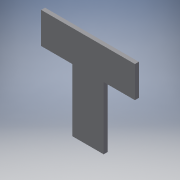
# Autodesk Inventor part: Frame T Gussets
Saved by Autodesk Inventor 2017 (Build 210142000, 142)
## iProperties
Created: 2017-12-29
Part Number: Frame T Gussets
Material: Generic
Document SubType Name: Modeling
Designer: anikasoojin
Density: 1 g/cm^3
Appearance: Default
Author: anikasoojin
Autodesk Inventor part; units mm, degrees
ref_plane "YZ Plane" through (0, 0, 0) normal (1, 0, 0) x (0, 1, 0)
ref_plane "XZ Plane" through (0, 0, 0) normal (0, 1, 0) x (-1, 0, 0)
ref_plane "XY Plane" through (0, 0, 0) normal (0, 0, 1) x (1, 0, 0)
sketch "Sketch1" plane through (0, 0, 0) normal (0, 0, 1) x (1, 0, 0)
  line L0 (-18.0361, 37.9933) -> (2.0277, 37.9933)
  line L1 (6.0832, 12.5933) -> (6.0832, -38.2067)
  line L2 (6.0832, -38.2067) -> (-19.3168, -38.2067)
  line L3 (-19.3168, -38.2067) -> (-19.3168, 12.5933)
  line L4 (-44.7168, 37.9933) -> (31.4832, 37.9933)
  line L5 (31.4832, 37.9933) -> (31.4832, 12.5933)
  line L6 (-44.7168, 12.5933) -> (-44.7168, 37.9933)
  line L7 (31.4832, 12.5933) -> (6.0832, 12.5933)
  line L8 (-19.3168, 12.5933) -> (-44.7168, 12.5933)
  point P0 (0, 0)
  dimension "d0" = 76.2
  dimension "d1" = 25.4
  dimension "d2" = 25.4
  dimension "d3" = 25.4
  dimension "d4" = 50.8
  dimension "d5" = 25.4
  constraints: 18 end point, 5 parallel, 2 horizontal, 2 perpendicular, 1 point on line
  measures "d0" distance between parallel lines of L5 L6
  measures "d1" distance of L1.end L2.end
  measures "d2" distance of L4.end L5.end
  measures "d3" distance of L6.start L4.start
  measures "d4" distance of L1.start L1.end
  measures "d5" distance of L3.end L6.start
extrude "Extrusion1" add sketch "Sketch1" along normal blind 3.175
fillet "Fillet1" radius 3.175 3 edges at (-44.7168, 12.5933, 1.5875) (-19.3168, 12.5933, 1.5875) (-19.3168, -38.2067, 1.5875)
fillet "Fillet2" radius 3.175 1 edges at (6.0832, -38.2067, 1.5875)
fillet "Fillet3" radius 3.175 3 edges at (6.0832, 12.5933, 1.5875) (31.4832, 12.5933, 1.5875) (31.4832, 37.9933, 1.5875)
fillet "Fillet4" radius 3.175 1 edges at (-44.7168, 37.9933, 1.5875)
sketch "Sketch2" plane through (0, 0, 3.175) normal (0, 0, 1) x (1, 0, 0)
  line L0 (31.4832, 15.7683) -> (31.4832, 34.8183) projected
  line L1 (31.4832, 25.2933) -> (-44.7168, 25.2933) construction
  line L2 (-44.7168, 34.8183) -> (-44.7168, 15.7683) projected
  line L3 (28.3082, 37.9933) -> (-41.5418, 37.9933) projected
  line L4 (-6.6168, 37.9933) -> (-6.6168, -38.2067) construction
  line L5 (-16.1418, -38.2067) -> (2.9082, -38.2067) projected
  circle A0 centre (18.7832, 25.2933) radius 3.175
  circle A1 centre (-6.6168, 25.2933) radius 3.175
  circle A2 centre (-32.0168, 25.2933) radius 3.175
  circle A3 centre (-6.6168, -0.1067) radius 3.175
  circle A4 centre (-6.6168, -25.5067) radius 3.175
  point P0 (0, 0)
  dimension "d12" = 6.35
  dimension "d13" = 12.7
  dimension "d16" = 25.4
  dimension "d23" = 25.4
  constraints: 5 centre point, 4 end point, 4 midpoint, 1 horizontal, 1 point on line, 1 vertical, 8 other
  measures "d12" diameter of A0
  measures "d13" distance of L1.start A0.centre
  measures "d16" distance of A0.centre A1.centre
  measures "d23" distance of A1.centre A3.centre
extrude "Extrusion2" cut sketch "Sketch2" against normal through all
body "Solid1"
